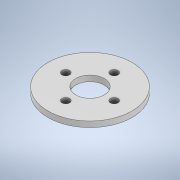
# Autodesk Inventor part: Inner_flange
Saved by Autodesk Inventor 2020.4 (Build 244396000, 396)
## iProperties
Part Number: Inner_flange
Material: アルミニウム 2014-T4
Document SubType Name: Modeling
Designer: Masato Kubotera
Density: 2.8 g/cm^3
Appearance: 滑らか - 淡い灰色
Mass: 2.85379 g
Surface Area: 13.2533 cm^2
Volume: 1.01921 cm^3
Description: A2017 T2
Author: Masato Kubotera
Autodesk Inventor part; units mm, degrees
ref_plane "YZ Plane" through (0, 0, 0) normal (1, 0, 0) x (0, 1, 0)
ref_plane "XZ Plane" through (0, 0, 0) normal (0, 1, 0) x (-1, 0, 0)
ref_plane "XY Plane" through (0, 0, 0) normal (0, 0, 1) x (1, 0, 0)
sketch "スケッチ1" plane through (0, 0, 0) normal (0, 0, 1) x (1, 0, 0)
  circle A0 centre (0, 0) radius 14.75
  line L0 (0, 14.75) -> (0, -14.75) construction
  circle A1 centre (0, 8.5) radius 1.35
  circle A2 centre (-8.5, 0) radius 1.35
  circle A3 centre (0, -8.5) radius 1.35
  circle A4 centre (8.5, 0) radius 1.35
  circle A5 centre (0, 0) radius 5 construction
  circle A6 centre (0, 0) radius 5.01
  dimension "d0" = 29.5
  dimension "d1" = 2.7
  dimension "d2" = 8.5
  dimension "d5" = 360
  dimension "d7" = 10
  dimension "d8" = 0.01
  constraints: 7 centre point, 3 coincident, 2 end point, 2 point on circle, 1 midpoint, 1 point on line, 1 vertical, 9 other
  measures "d0" diameter of A0
  measures "d1" diameter of A1
  measures "d2" distance of point (0, 0) A1.centre
  measures "d7" diameter of A5
  measures "d8" radial gap between concentric circles of A6 A5
extrude "押し出し1" add sketch "スケッチ1" along normal blind 2
